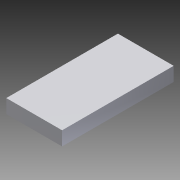
# Autodesk Inventor part: IOIO
Saved by Autodesk Inventor 2014 (Build 180170000, 170)
## iProperties
Created: 2014-04-26
Part Number: IOIO
Material: Generic
Document SubType Name: Modeling
Designer: dclar4
Density: 1 g/cm^3
Appearance: Snow
Author: dclar4
Autodesk Inventor part; units mm, degrees
ref_plane "YZ Plane" through (0, 0, 0) normal (1, 0, 0) x (0, 1, 0)
ref_plane "XZ Plane" through (0, 0, 0) normal (0, 1, 0) x (-1, 0, 0)
ref_plane "XY Plane" through (0, 0, 0) normal (0, 0, 1) x (1, 0, 0)
sketch "Sketch1" plane through (0, 0, 0) normal (0, 1, 0) x (-1, 0, 0)
  line L0 (-10.7162, 11.6704) -> (40.0838, 11.6704)
  line L1 (40.0838, 11.6704) -> (40.0838, -89.9296)
  line L2 (40.0838, -89.9296) -> (-10.7162, -89.9296)
  line L3 (-10.7162, -89.9296) -> (-10.7162, 11.6704)
  point P0 (0, 0)
  dimension "d0" = 50.8
  dimension "d1" = 101.6
  constraints: 8 end point, 2 parallel, 1 horizontal, 1 perpendicular
  measures "d0" distance of L1.end L2.end
  measures "d1" distance of L0.end L1.end
extrude "Extrusion1" add sketch "Sketch1" along normal blind 12.7
body "Solid1"
